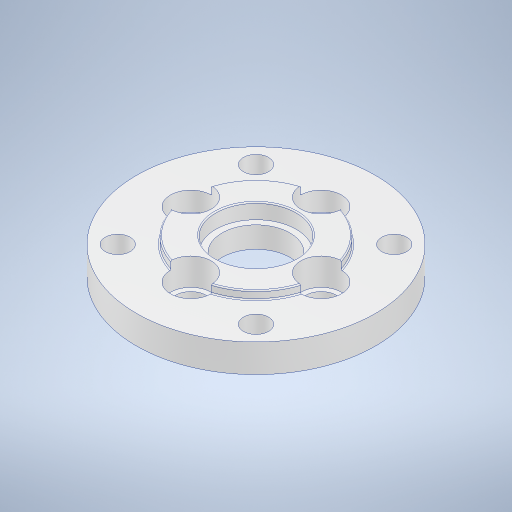
# Autodesk Inventor part: Motor Plate
Saved by Autodesk Inventor 2023.2 (Build 272271000, 271)
## iProperties
Created: 2023-01-20
Part Number: Motor Plate
Material: Aluminum 6061
Document SubType Name: Modeling
Designer: Nathan Cai
Density: 2.7 g/cm^3
Appearance: Aluminum - Flat
Author: Nathan Cai
Autodesk Inventor part; units mm, degrees
ref_plane "YZ Plane" through (0, 0, 0) normal (1, 0, 0) x (0, 1, 0)
ref_plane "XZ Plane" through (0, 0, 0) normal (0, 1, 0) x (-1, 0, 0)
ref_plane "XY Plane" through (0, 0, 0) normal (0, 0, 1) x (1, 0, 0)
sketch "Sketch1" plane through (0, 0, 0) normal (0, 1, 0) x (-1, 0, 0)
  circle A0 centre (0, 0) radius 11
  circle A1 centre (0, 0) radius 3.125
  dimension "d0" = 22
  dimension "d1" = 6.25
  constraints: 2 centre point, 2 coincident
  measures "d0" diameter of A0
  measures "d1" diameter of A1
extrude "Extrusion1" add sketch "Sketch1" along normal blind 2.6
sketch "Sketch2" plane through (0, 2.6, 0) normal (0, 1, 0) x (1, 0, 0)
  circle A0 centre (0, 0) radius 6.25
  circle A1 centre (0, 0) radius 3.125
  dimension "d4" = 12.5
  constraints: 2 centre point, 2 coincident
  measures "d4" diameter of A0
extrude "Extrusion2" add sketch "Sketch2" along normal blind 0.75
sketch "Sketch3" plane through (0, 3.35, 0) normal (0, 1, 0) x (1, 0, 0)
  circle A0 centre (0, 0) radius 3.7
  dimension "d7" = 7.4
  constraints: 1 centre point, 1 coincident
  measures "d7" diameter of A0
extrude "Extrusion3" cut sketch "Sketch3" against normal blind 1.4
sketch "Sketch4" plane through (0, 2.6, 0) normal (0, 1, 0) x (1, 0, 0)
  circle A0 centre (0, 0) radius 11 construction
  line L0 (0, 0) -> (-11, 0)
  circle A1 centre (0, 0) radius 11 projected
  circle A2 centre (-6, 0) radius 1.4
  circle A3 centre (0, -6) radius 1.4
  circle A4 centre (6, 0) radius 1.4
  circle A5 centre (0, 6) radius 1.4
  dimension "d10" = 22
  dimension "d11" = 2.8
  dimension "d12" = 6
  dimension "d15" = 360
  constraints: 5 centre point, 2 end point, 1 coincident, 1 horizontal, 1 horizontal alignment, 1 point on line, 10 other
  measures "d10" diameter of A0
  measures "d11" diameter of A2
  measures "d12" distance of point (0, 0) A2.centre
extrude "Extrusion4" cut sketch "Sketch4" along normal through all both and the other way through all contours A2 L0 | L0 A2 | A3 | A4 | A5
sketch "Sketch5" plane through (0, 3.35, 0) normal (0, 1, 0) x (1, 0, 0)
  circle A0 centre (-6, 0) radius 1.4 projected
  circle A1 centre (-6, 0) radius 1.875
  circle A2 centre (0, -6) radius 1.875
  circle A3 centre (6, 0) radius 1.875
  circle A4 centre (0, 6) radius 1.875
  point P0 (0, 0)
  dimension "d19" = 3.75
  dimension "d22" = 360
  constraints: 4 centre point, 1 coincident, 9 other
  measures "d19" diameter of A1
extrude "Extrusion5" cut sketch "Sketch5" against normal blind 2.5 contours A0 | A1 | A2 | A3 | A4
sketch "Sketch6" plane through (0, 2.6, 0) normal (0, 1, 0) x (1, 0, 0)
  line L0 (0, 0) -> (-7.7782, -7.7782) construction
  circle A0 centre (0, 0) radius 11 projected
  line L1 (0, 0) -> (11, 0) construction
  circle A1 centre (0, 0) radius 9 construction
  circle A2 centre (-6.364, -6.364) radius 1.15
  circle A3 centre (6.364, -6.364) radius 1.15
  circle A4 centre (6.364, 6.364) radius 1.15
  circle A5 centre (-6.364, 6.364) radius 1.15
  dimension "d27" = 18
  dimension "d26" = 135
  dimension "d28" = 2.3
  dimension "d31" = 360
  constraints: 4 centre point, 4 end point, 1 coincident, 1 equal length, 1 horizontal, 1 point on line, 14 other
  measures "d26" angle of L0 L1
  measures "d28" diameter of A2
extrude "Extrusion6" cut sketch "Sketch6" against normal through all contours A2 | A3 | A4 | A5
fillet "Fillet1" radius 0.1 9 edges at (-3.7, 3.35, 0) (-4.4194, 3.35, 4.4194) (-4.4194, 3.35, -4.4194) (4.4194, 3.35, -4.4194) (4.4194, 3.35, 4.4194) (4.4194, 2.6, 4.4194) (4.4194, 2.6, -4.4194) (-4.4194, 2.6, 4.4194) (-4.4194, 2.6, -4.4194)
body "Solid1"
